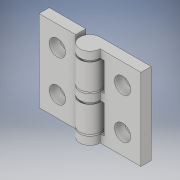
# Autodesk Inventor part: 26.2 scharnier 0.3 mm speling
Saved by Autodesk Inventor 2019 (Build 230136000, 136)
## iProperties
Created: 2021-01-06
Part Number: 26.2 scharnier 0.3 mm speling
Material: Generic
Document SubType Name: Modeling
Designer: semboonen
Density: 1 g/cm^3
Appearance: Default
Author: semboonen
Autodesk Inventor part; units mm, degrees
ref_plane "YZ Plane" through (0, 0, 0) normal (1, 0, 0) x (0, 1, 0)
ref_plane "XZ Plane" through (0, 0, 0) normal (0, 1, 0) x (-1, 0, 0)
sketch "Sketch1" plane through (0, 0, 0) normal (0, 0, 1) x (1, 0, 0)
  line L0 (12.5, -10) -> (12.5, 10)
  line L1 (-12.5, 10) -> (-12.5, -10)
  line L2 (-12.5, -10) -> (12.5, 10) construction
  line L3 (12.5, -10) -> (-12.5, 10) construction
  line L4 (2.5, -10) -> (2.5, 10)
  line L5 (-2.5, 10) -> (-2.5, -10)
  line L6 (-2.5, -10) -> (2.5, 10) construction
  line L7 (2.5, -10) -> (-2.5, 10) construction
  line L8 (12.5, 10) -> (2.5, 10)
  line L9 (-2.5, 10) -> (-12.5, 10)
  line L10 (-12.5, -10) -> (-2.5, -10)
  line L11 (2.5, -10) -> (12.5, -10)
  point P0 (0, 0)
  dimension "d0" = 25
  dimension "d1" = 20
  dimension "d2" = 5
  dimension "d3" = 20
  dimension "d4" = 38.66
  dimension "d5" = 75.964
  constraints: 24 end point, 4 equal length, 4 midpoint, 1 horizontal, 1 vertical
  measures "d0" distance of L1.start L0.end
  measures "d1" distance of L0.start L0.end
  measures "d2" distance of L5.start L4.end
  measures "d3" distance of L4.end L4.start
  measures "d4" angle of L8 L3
  measures "d5" angle of L11 L6
extrude "Extrusion1" add sketch "Sketch1" along normal blind 2.5
sketch "Sketch2" plane through (0, 0, 2.5) normal (0, 0, 1) x (1, 0, 0)
  line L0 (-2.5, -10) -> (-2.5, 10) projected
  line L1 (12.5, 10) -> (2.5, 10) projected
  line L2 (-2.5, 10) -> (0, 10)
  line L3 (2.5, 10) -> (2.5, -10) projected
  line L4 (-2.5, 10) -> (-2.5, 8.0707)
  line L5 (0, 5.5707) -> (0, 10)
  line L6 (-2.5, 7.75) -> (1.5, 7.75) construction
  line L7 (-2.5, 0) -> (-2.5, 1)
  line L8 (0, 0) -> (0, 3.5)
  line L9 (-2.5, 1) -> (-2.5, 1.25) construction
  line L10 (0, 3.75) -> (0, 5.1793)
  line L11 (-2.5, 1.25) -> (-2.5, 7.6793)
  line L12 (-2.5, -10) -> (0, -10)
  line L13 (-2.5, -10) -> (-2.5, -8.0707)
  line L14 (0, -5.5707) -> (0, -10)
  line L15 (-2.5, 0) -> (-2.5, -0.9293)
  line L16 (0, 0) -> (0, -3.4293)
  line L17 (-2.5, -1) -> (-2.5, -1.25) construction
  line L18 (0, -3.8207) -> (0, -5.1793)
  line L19 (-2.5, -1.3207) -> (-2.5, -7.6793)
  line L20 (0, -5.5707) -> (-2.5, -8.0707)
  line L21 (0, -5.1793) -> (-2.5, -7.6793)
  line L22 (0, -3.8207) -> (-2.5, -1.3207)
  line L23 (0, -3.4293) -> (-2.5, -0.9293)
  line L24 (0, 3.8207) -> (-2.5, 1.3207)
  line L25 (0, 5.1793) -> (-2.5, 7.6793)
  line L26 (0, 5.5707) -> (-2.5, 8.0707)
  line L27 (-2.5, 0.9293) -> (0, 3.4293)
  point P0 (-2.5, 8)
  dimension "d11" = 2
  dimension "d15" = 1
  dimension "d18" = 0.25
  dimension "d19" = 90
  dimension "d20" = 90
  dimension "d21" = 90
  dimension "d22" = 90
  dimension "d23" = 90
  dimension "d24" = 90
  dimension "d25" = 90
  dimension "d26" = 2.5
  dimension "d27" = 2.25
  dimension "d28" = 2.5
  dimension "d33" = 12.5
  dimension "d34" = 12.5
  dimension "d35" = 1
  dimension "d73" = 45
  dimension "d74" = 90
  dimension "d75" = 6.364
  dimension "d76" = 6.6407
  dimension "d77" = 0.2768
  dimension "d78" = 6.364
  dimension "d79" = 6.0872
  dimension "d80" = 0.2768
  dimension "d81" = 4.4694
  dimension "d82" = 12.2476
  dimension "d83" = 15
  dimension "d84" = 15
  dimension "d85" = 6.25
  dimension "d86" = 6.5
  dimension "d87" = 11
  dimension "d88" = 11.25
  constraints: 50 end point, 9 parallel, 8 point on line, 2 horizontal, 1 collinear, 1 midpoint, 1 perpendicular, 1 vertical
  measures "d11" distance of L0.end point (-2.5, 8)
  measures "d15" distance of L7.start L7.end
  measures "d18" distance of L7.end L9.end
  measures "d19" angle of L1 L8
  measures "d20" angle of L1 L16
  measures "d21" angle of L1 L18
  measures "d22" angle of L1 L15
  measures "d23" angle of L1 L17
  measures "d24" angle of L1 L19
  measures "d25" angle of L5 L1
  measures "d26" distance between parallel lines of L3 L10
  measures "d27" distance between parallel lines of L6 L1
  measures "d28" distance between parallel lines of L14 L3
  measures "d33" distance from line of L1.start L5
  measures "d34" distance from line of L1.start L18
  measures "d35" distance from line of L6.end L3
  measures "d73" angle of L1 L20
  measures "d74" angle of L4 L1
  measures "d75" distance between parallel lines of L24 L21
  measures "d76" distance between parallel lines of L24 L20
  measures "d77" distance between parallel lines of L24 L27
  measures "d78" distance between parallel lines of L25 L22
  measures "d79" distance between parallel lines of L25 L23
  measures "d80" distance between parallel lines of L26 L25
  measures "d81" distance from line of L1.start L24
  measures "d82" distance from line of L1.start L25
  measures "d83" distance from line of L1.start L17
  measures "d84" distance from line of L1.start L19
  measures "d85" distance from line of L10.start L1
  measures "d86" distance from line of L8.end L1
  measures "d87" distance from line of L17.start L1
  measures "d88" distance from line of L17.end L1
revolve "Revolution1" add sketch "Sketch2" angle 360 about axis through (0, 0, 2.5) along (0, 1, 0)
sketch "Sketch4" plane through (0, 0, 2.5) normal (0, 0, 1) x (1, 0, 0)
  line L0 (-2.5, -1.3207) -> (-2.5, 8.0707) projected
  line L1 (-2.5, 7.75) -> (-3.5, 7.75)
  line L2 (-3.5, 7.75) -> (-3.5, 10)
  line L3 (-3.5, 10) -> (-2.5, 10)
  line L4 (-2.5, 10) -> (-2.5, 7.75)
  line L5 (2.5, 10) -> (2.5, 8.0707) projected
  line L6 (2.5, 8) -> (3.5, 8)
  line L7 (3.5, 8) -> (3.5, 1)
  line L8 (3.5, 1) -> (2.5, 1)
  line L9 (2.5, 1) -> (2.5, 8)
  line L10 (-2.5, -7.6793) -> (-2.5, -1.3207) projected
  line L11 (-2.5, -1.25) -> (-3.5, -1.25)
  line L12 (-3.5, -1.25) -> (-3.5, 1.25)
  line L13 (-3.5, 1.25) -> (-2.5, 1.25)
  line L14 (-2.5, 1.25) -> (-2.5, -1.25)
  line L15 (2.5, 0.9293) -> (2.5, -0.9293) projected
  line L16 (2.5, -1) -> (3.5, -1)
  line L17 (3.5, -1) -> (3.5, -8)
  line L18 (3.5, -8) -> (2.5, -8)
  line L19 (2.5, -8) -> (2.5, -1)
  line L20 (2.5, -7.6793) -> (-2.5, -7.6793) projected
  line L21 (-2.5, -10) -> (-12.5, -10) projected
  line L22 (-2.5, -7.6793) -> (-3.5, -7.6793)
  line L23 (-3.5, -7.6793) -> (-3.5, -10)
  line L24 (-3.5, -10) -> (-2.5, -10)
  line L25 (-2.5, -10) -> (-2.5, -7.6793)
  point P0 (0, 0)
  point P1 (-2.5, 8)
  point P2 (0, -7.6793)
  dimension "d39" = 1
  dimension "d40" = 2.25
  dimension "d41" = 1
  dimension "d42" = 7
  dimension "d43" = 1
  dimension "d44" = 2.5
  dimension "d45" = 1
  dimension "d46" = 7
  dimension "d47" = 1
  constraints: 40 end point, 10 parallel, 5 horizontal, 5 perpendicular, 1 point on line
  measures "d39" distance of L2.end L3.end
  measures "d40" distance of L1.end L2.end
  measures "d41" distance of L7.end L8.end
  measures "d42" distance of L6.end L7.end
  measures "d43" distance of L12.end L13.end
  measures "d44" distance of L11.end L12.end
  measures "d45" distance of L17.end L18.end
  measures "d46" distance of L16.end L17.end
  measures "d47" distance of L24.end L23.end
extrude "Extrusion3" cut sketch "Sketch4" against normal blind 2.5
sketch "Sketch5" plane through (0, 0, 2.5) normal (0, 0, 1) x (1, 0, 0)
  circle A0 centre (8, -5) radius 2
  line L0 (2.5, -10) -> (12.5, -10) projected
  line L1 (12.5, -10) -> (12.5, 10) projected
  line L2 (-12.5, 10) -> (-12.5, -10) projected
  line L3 (-12.5, -10) -> (-3.5, -10) projected
  circle A1 centre (8, 5) radius 2
  circle A2 centre (-8, -5) radius 2
  circle A3 centre (-8, 5) radius 2
  point P0 (0, 0)
  dimension "d50" = 4
  dimension "d51" = 5
  dimension "d52" = 4.5
  dimension "d57" = 10
  dimension "d60" = 16
  constraints: 4 centre point, 1 horizontal, 1 vertical, 6 other
  measures "d50" diameter of A0
  measures "d51" distance from line of L0 A0.centre
  measures "d52" distance from line of L1 A0.centre
  measures "d57" distance of A0.centre A1.centre
  measures "d60" distance of A0.centre A2.centre
extrude "Extrusion4" cut sketch "Sketch5" against normal blind 2.5
sketch "Sketch6" plane through (0, 0, 0) normal (0, 0, -1) x (-1, 0, 0)
  line L0 (-2.5, 8) -> (-2.5, 10) projected
  line L1 (2.5, 8.0707) -> (-2.5, 8.0707) projected
  line L2 (-2.5, 10) -> (0, 10)
  line L3 (0, 10) -> (0, 8.0707)
  line L4 (0, 8.0707) -> (-2.5, 8.0707)
  line L5 (-2.5, 8.0707) -> (-2.5, 10)
  line L6 (2.5, 7.6793) -> (0, 5.1793) projected
  line L7 (2.5, 1.25) -> (3.5, 1.25) projected
  line L8 (-2.5, 0.9293) -> (-2.5, -0.9293) projected
  line L9 (2.5, -0.9293) -> (-2.5, -0.9293) projected
  line L10 (-2.5, 0.9293) -> (0, 0.9293)
  line L11 (0, 0.9293) -> (0, -0.9293)
  line L12 (0, -0.9293) -> (-2.5, -0.9293)
  line L13 (-2.5, -0.9293) -> (-2.5, 0.9293)
  line L14 (-2.5, -8.0707) -> (-2.5, -10) projected
  line L15 (2.5, -8.0707) -> (-2.5, -8.0707) projected
  line L16 (-2.5, -10) -> (0, -10)
  line L17 (0, -10) -> (0, -8.0707)
  line L18 (0, -8.0707) -> (-2.5, -8.0707)
  line L19 (-2.5, -8.0707) -> (-2.5, -10)
  line L20 (0, 3.8207) -> (2.5, 1.3207) projected
  line L21 (0, -5.1793) -> (-2.5, -7.6793) projected
  line L22 (-2.5, -1.3207) -> (0, -3.8207) projected
  line L23 (0, -3.8207) -> (0, -5.1793)
  line L24 (0, -5.1793) -> (2.5, -7.6793) projected
  line L25 (0, 5.1793) -> (2.5, 5.1793)
  line L26 (2.5, 7.75) -> (2.5, 1.25) projected
  line L27 (0, 3.8207) -> (2.5, 3.8207)
  line L28 (2.5, 3.8207) -> (2.5, 5.1793)
  line L29 (0, -3.8207) -> (2.5, -3.8207)
  line L30 (2.5, -1.25) -> (2.5, -7.6793) projected
  line L31 (0, -5.1793) -> (2.5, -5.1793)
  line L32 (2.5, -3.8207) -> (2.5, -5.1793)
  line L33 (0, 5.1793) -> (0, 3.8207)
  point P0 (0, 0)
  point P1 (2.5, -1.3207)
  constraints: 40 end point, 7 parallel, 6 horizontal, 6 perpendicular, 4 point on line, 3 midpoint, 1 vertical
extrude "Extrusion5" add sketch "Sketch6" against normal blind 2.5 contours L0 L2 L3 L1 | L25 L26 L27 L33 | L10 L11 L9 L8 | L15 L17 L16 L14 | L29 L30 L31 L23
sketch "Sketch7" plane through (-2.5, -5.1793, 0) normal (0, -1, 0) x (1, 0, 0)
  line L0 (2.5, 0) -> (0, 0)
  circle A0 centre (2.5, 2.5) radius 2.5 projected
  line L1 (0, 0) -> (0, 2.5) projected
  line L2 (0, 0) -> (0, 2.5)
  line L3 (-1, 2.5) -> (0, 2.5) projected
  arc A1 (0, 2.5) -> (2.5, 0) centre (2.5, 2.5) ccw
  constraints: 4 end point, 2 concentric, 2 point on circle, 1 centre point, 1 collinear, 1 horizontal, 1 tangent
extrude "Extrusion6" add sketch "Sketch7" along normal blind 2.5 contours L0 L1 A0
sketch "Sketch8" plane through (-2.5, -3.8207, 0) normal (0, 1, 0) x (1, 0, 0)
  line L0 (0, -2.5) -> (-1, -2.5) projected
  line L1 (0, 0) -> (2.5, 0) projected
  line L2 (0, -2.5) -> (0, 0)
  line L3 (0, 0) -> (2.5, 0)
  line L4 (0, 0) -> (0, -2.5) projected
  arc A0 (2.5, 0) -> (0, -2.5) centre (2.5, -2.5) ccw
  constraints: 4 end point, 2 point on circle, 1 centre point, 1 collinear, 1 tangent, 1 vertical
extrude "Extrusion7" add sketch "Sketch8" along normal blind 2.5
ref_plane "Work Plane1" through (-2.5, 4.5, 0) normal (0, 1, 0) x (1, 0, 0)
sketch "Sketch9" plane through (-2.5, 4.5, 0) normal (0, 1, 0) x (1, 0, 0)
  line L0 (0, -2.5) -> (-1, -2.5) projected
  line L1 (0, -2.5) -> (0, 0) projected
  line L2 (0, -2.5) -> (0, 0)
  line L3 (2.5, 0) -> (0, 0) projected
  line L4 (0, 0) -> (2.5, 0)
  arc A0 (2.5, 0) -> (0, -2.5) centre (2.5, -2.5) ccw
  constraints: 4 end point, 2 point on circle, 2 tangent, 1 centre point, 1 collinear, 1 vertical
extrude "Extrusion8" add sketch "Sketch9" along normal mid plane 6.35
body "Solid1"
